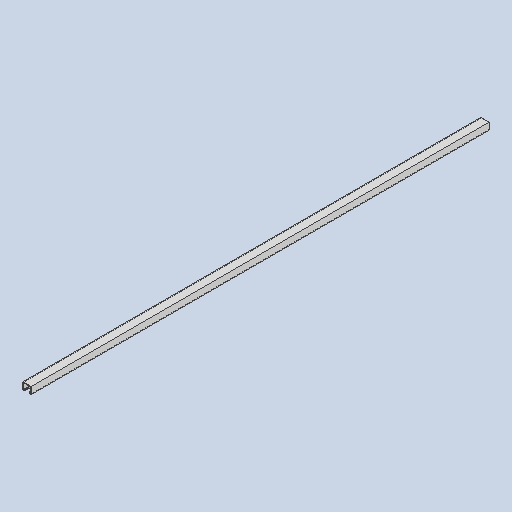
# Autodesk Inventor part: LongStrut84Sec1
Saved by Autodesk Inventor 2023 (Build 270158030, 158C)
## iProperties
Created: 2022-06-29
Part Number: LongStrut84Sec1
Material: Generic
Document SubType Name: Modeling
Designer: jeremyy
Density: 1 g/cm^3
Appearance: Default
Author: jeremyy
Autodesk Inventor part; units mm, degrees
ref_plane "YZ Plane" through (0, 0, 0) normal (1, 0, 0) x (0, 1, 0)
ref_plane "XZ Plane" through (0, 0, 0) normal (0, 1, 0) x (-1, 0, 0)
ref_plane "XY Plane" through (0, 0, 0) normal (0, 0, 1) x (1, 0, 0)
sketch "Sketch1" plane through (0, 0, 0) normal (0, 0, 1) x (1, 0, 0)
  line L0 (0, 0) -> (41.275, 0)
  line L1 (41.275, 0) -> (41.275, -34.925)
  line L2 (41.275, -34.925) -> (31.75, -34.925)
  line L3 (31.75, -34.925) -> (31.75, -27.7812)
  line L4 (31.75, -27.7812) -> (34.35, -27.7812)
  line L5 (34.35, -27.7812) -> (34.35, -32.325)
  line L6 (34.35, -32.325) -> (38.675, -32.325)
  line L7 (38.675, -32.325) -> (38.675, -2.6)
  line L8 (38.675, -2.6) -> (2.6, -2.6)
  line L9 (0, -34.925) -> (0, 0)
  line L10 (2.6, -2.6) -> (2.6, -32.325)
  line L11 (2.6, -32.325) -> (6.7091, -32.325)
  line L12 (6.7091, -32.325) -> (6.7091, -27.7812)
  line L13 (6.7091, -27.7812) -> (9.3091, -27.7812)
  line L14 (9.3091, -27.7812) -> (9.3091, -34.925)
  line L15 (9.3091, -34.925) -> (0, -34.925)
  dimension "d0" = 41.275
  dimension "d1" = 34.925
  dimension "d4" = 9.525
  dimension "d5" = 7.1437
  dimension "d6" = 2.6
  dimension "d7" = 2.6
  dimension "d8" = 2.6
  dimension "d9" = 2.6
  dimension "d11" = 2.6
  dimension "d12" = 2.6
  dimension "d13" = 7.1437
  dimension "d14" = 2.6
  constraints: 32 end point, 13 perpendicular, 2 horizontal, 1 point on line, 1 vertical
  measures "d0" distance of L0.start L0.end
  measures "d1" distance of L0.end L1.end
  measures "d4" distance of L1.end L2.end
  measures "d5" distance of L2.end L3.end
  measures "d6" distance of L3.end L4.end
  measures "d7" distance between parallel lines of L2 L6
  measures "d8" distance between parallel lines of L1 L7
  measures "d9" distance between parallel lines of L8 L0
  measures "d11" distance between parallel lines of L15 L11
  measures "d12" distance between parallel lines of L14 L12
  measures "d13" distance of L13.end L14.end
  measures "d14" distance between parallel lines of L10 L9
extrude "Extrusion1" add sketch "Sketch1" along normal blind 2286
body "Solid1"
